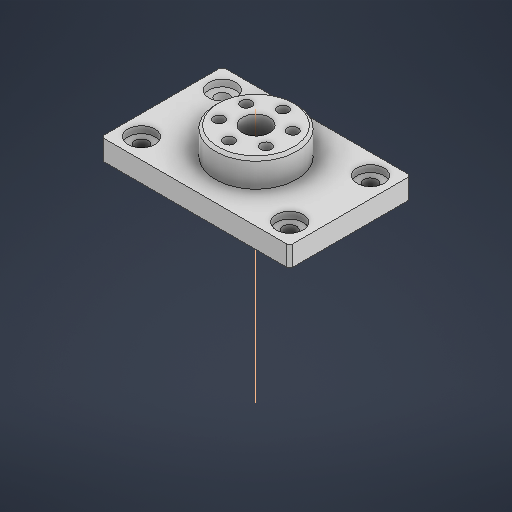
# Autodesk Inventor part: desticka
Saved by Autodesk Inventor 2026 (Build 300175000, 175)
## iProperties
Created: 2025-05-26
Part Number: desticka
Material: Všeobecné
Document SubType Name: Modeling
Designer: daniel
Density: 1 g/cm^3
Appearance: Výchozí
Author: daniel
Autodesk Inventor part; units mm, degrees
ref_plane "YZ Plane" through (0, 0, 0) normal (1, 0, 0) x (0, 1, 0)
ref_plane "XZ Plane" through (0, 0, 0) normal (0, 1, 0) x (-1, 0, 0)
ref_plane "XY Plane" through (0, 0, 0) normal (0, 0, 1) x (1, 0, 0)
sketch "Náčrt3" plane through (0, 0, 0) normal (0, 1, 0) x (-1, 0, 0)
  line L0 (-70, 45) -> (70, 45)
  line L1 (70, 45) -> (70, -45)
  line L2 (70, -45) -> (-70, -45)
  line L3 (-70, -45) -> (-70, 45)
  line L4 (-70, 45) -> (70, -45) construction
  line L5 (70, 45) -> (-70, -45) construction
  point P0 (0, 0)
  dimension "d31" = 140
  dimension "d32" = 90
  constraints: 12 end point, 2 midpoint, 2 parallel, 1 horizontal, 1 perpendicular
  measures "d31" distance of L1.end L2.end
  measures "d32" distance of L0.end L1.end
extrude "Vysunutí2" add sketch "Náčrt3" along normal blind 15
chamfer "Zkosení5" distance 2 angle 45 1 edges at (70, 7.5, 45)
chamfer "Zkosení6" distance 2 angle 45 1 edges at (70, 7.5, -45)
chamfer "Zkosení7" distance 2 angle 45 1 edges at (-70, 7.5, 45)
chamfer "Zkosení8" distance 2 angle 45 1 edges at (-70, 7.5, -45)
sketch "Náčrt4" plane through (0, 15, 0) normal (0, 1, 0) x (1, 0, 0)
  line L0 (68, 45) -> (-68, 45) projected
  line L1 (-70, 43) -> (-70, -43) projected
  point P0 (0, 0)
  point P1 (-55, 30)
  dimension "d47" = 15
  dimension "d48" = 15
  measures "d47" distance from line of L0 point (-55, 30)
  measures "d48" distance from line of L1 point (-55, 30)
hole "Díra2" at (-55, 15, -30) direction (0, -1, 0) diameter 10 end through all counterbore diameter 20 counterbore depth 5
pattern_linear "Obdélníkové pole2" count 2 spacing 110 along (1, 0, 0) count 2 spacing 60 along (0, 0, 1) of "Díra2"
sketch "Náčrt5" plane through (0, 15, 0) normal (0, 1, 0) x (1, 0, 0)
  circle A0 centre (0, 0) radius 30
  dimension "d62" = 60
  constraints: 1 centre point, 1 coincident
  measures "d62" diameter of A0
extrude "Vysunutí3" add sketch "Náčrt5" along normal blind 20
chamfer "Zkosení9" distance 2 angle 45 1 edges at (-30, 35, 0)
sketch "Náčrt6" plane through (0, 35, 0) normal (0, 1, 0) x (1, 0, 0)
  circle A0 centre (0, 0) radius 28 projected
  constraints: 1 coincident
hole "Díra3" at (0, 35, 0) direction (0, -1, 0) diameter 20 end through all
sketch "Náčrt12" plane through (0, 35, 0) normal (0, 1, 0) x (1, 0, 0)
  circle A0 centre (0, 0) radius 20
  circle A1 centre (0, 20) radius 4
  dimension "d114" = 40
  dimension "d115" = 8
  constraints: 1 centre point, 1 coincident, 1 vertical alignment, 2 other
  measures "d115" diameter of A1
extrude "Vysunutí4" cut sketch "Náčrt12" against normal through all contours A1 A0 | A0 A1 picked at (0, 18.6369) picked at (0.0994, 21.2999)
pattern_circular "Kruhové pole2" count 6 over 360 about axis through (0, -135.0735, 0) along (0, 1, 0) of "Vysunutí4"
